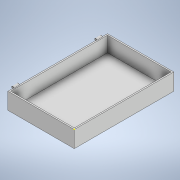
# Autodesk Inventor part: chestLower
Saved by Autodesk Inventor 2020.3 (Build 243373000, 373)
## iProperties
Created: 2021-02-24
Part Number: chestLower
Material: Generic
Document SubType Name: Modeling
Designer: con_c_000
Density: 1 g/cm^3
Appearance: Default
Author: con_c_000
Autodesk Inventor part; units mm, degrees
ref_plane "YZ Plane" through (0, 0, 0) normal (1, 0, 0) x (0, 1, 0)
ref_plane "XZ Plane" through (0, 0, 0) normal (0, 1, 0) x (-1, 0, 0)
ref_plane "XY Plane" through (0, 0, 0) normal (0, 0, 1) x (1, 0, 0)
sketch "Sketch1" plane through (0, 0, 0) normal (0, 1, 0) x (-1, 0, 0)
  line L0 (0, 0) -> (609.6, 0)
  line L1 (609.6, 0) -> (609.6, -914.4)
  line L2 (609.6, -914.4) -> (0, -914.4)
  line L3 (0, -914.4) -> (0, 0)
  dimension "d0" = 609.6
  dimension "d1" = 914.4
  constraints: 8 end point, 2 parallel, 1 horizontal, 1 perpendicular
  measures "d0" distance of L1.end L2.end
  measures "d1" distance of L0.end L1.end
extrude "Extrusion1" add sketch "Sketch1" along normal blind 152.4
shell "Shell1" thickness 12.7 removed faces 1 at (-203.2, 152.4, -304.8)
sketch "Sketch2" plane through (0, 0, -914.4) normal (0, 0, -1) x (-1, 0, 0)
  line L0 (596.9, 152.4) -> (12.7, 152.4) projected
  circle A0 centre (615.95, 152.4) radius 10.16
  circle A1 centre (615.95, 152.4) radius 6.35
  line L1 (609.6, 0) -> (609.6, 152.4) projected
  point P0 (0, 0)
  dimension "d5" = 12.7
  dimension "d6" = 20.32
  dimension "d7" = 6.35
  constraints: 2 centre point, 1 coincident, 1 point on line
  measures "d5" diameter of A1
  measures "d6" diameter of A0
  measures "d7" distance from line of L1 A1.centre
extrude "Extrusion2" add sketch "Sketch2" against normal up to surface (914.4 mm away)
sketch "Sketch3" plane through (0, 152.4, 0) normal (0, 1, 0) x (1, 0, 0)
  point P0 (0, 0)
sketch "Sketch4" plane through (0, 0, 0) normal (1, 0, 0) x (0, 0, -1)
  line L0 (0, 0) -> (0, 152.4) projected
  line L1 (0, 152.4) -> (50.8, 152.4)
  line L2 (50.8, 152.4) -> (50.8, 178.2149)
  line L3 (50.8, 178.2149) -> (0, 178.2149)
  line L4 (0, 178.2149) -> (0, 152.4)
  line L5 (914.4, 152.4) -> (863.6, 152.4)
  line L6 (863.6, 152.4) -> (863.6, 178.2149)
  line L7 (863.6, 178.2149) -> (914.4, 178.2149)
  line L8 (914.4, 178.2149) -> (914.4, 152.4)
  line L9 (0, 152.4) -> (914.4, 152.4) projected
  line L10 (101.6, 152.4) -> (812.8, 152.4)
  line L11 (812.8, 152.4) -> (812.8, 202.1874)
  line L12 (812.8, 202.1874) -> (101.6, 202.1874)
  line L13 (101.6, 202.1874) -> (101.6, 152.4)
  dimension "d10" = 50.8
  dimension "d11" = 50.8
  dimension "d12" = 50.8
  dimension "d13" = 50.8
  constraints: 24 end point, 6 parallel, 3 horizontal, 3 perpendicular, 2 point on line
  measures "d10" distance of L3.end L2.end
  measures "d11" distance of L6.end L7.end
  measures "d12" distance between parallel lines of L6 L11
  measures "d13" distance between parallel lines of L2 L13
extrude "Extrusion3" cut sketch "Sketch4" against normal through all
sketch "Sketch5" plane through (0, 152.4, 0) normal (0, 1, 0) x (1, 0, 0)
  line L0 (-609.6, 0) -> (-609.6, 914.4) projected
  line L1 (-609.6, 0) -> (-640.6567, 0)
  line L2 (-640.6567, 0) -> (-640.6567, 50.8)
  line L3 (-640.6567, 50.8) -> (-609.6, 50.8)
  line L4 (-609.6, 50.8) -> (-609.6, 0)
  line L5 (-609.6, 101.6) -> (-609.6, 812.8) projected
  line L6 (-609.6, 101.6) -> (-640.6567, 101.6)
  line L7 (-640.6567, 101.6) -> (-640.6567, 812.8)
  line L8 (-640.6567, 812.8) -> (-609.6, 812.8)
  line L9 (-609.6, 812.8) -> (-609.6, 101.6)
  line L10 (-609.6, 863.6) -> (-609.6, 914.4) projected
  line L11 (-609.6, 863.6) -> (-644.9488, 863.6)
  line L12 (-644.9488, 863.6) -> (-644.9488, 914.4)
  line L13 (-644.9488, 914.4) -> (-609.6, 914.4)
  line L14 (-609.6, 914.4) -> (-609.6, 863.6)
  point P0 (0, 0)
  constraints: 24 end point, 6 parallel, 3 horizontal, 3 perpendicular, 1 point on line
extrude "Extrusion4" cut sketch "Sketch5" against normal blind 25.4
body "Solid1"
